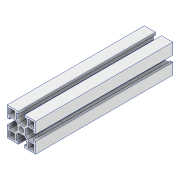
# Autodesk Inventor part: profile
Saved by Autodesk Inventor 2020 (Build 240168000, 168)
## iProperties
Created: 2020-09-09
Part Number: profile
Material: 알루미늄 6061
Document SubType Name: Modeling
Designer: 이호석
Mass: 133.418 g
Surface Area: 501.596 cm^2
Volume: 49.4139 cm^3
Density: 2.7 g/cm^3
Appearance: 알루미늄 - 평지
Author: 이호석
Autodesk Inventor part; units mm, degrees
ref_plane "YZ Plane" through (0, 0, 0) normal (1, 0, 0) x (0, 1, 0)
ref_plane "XZ Plane" through (0, 0, 0) normal (0, 1, 0) x (-1, 0, 0)
ref_plane "XY Plane" through (0, 0, 0) normal (0, 0, 1) x (1, 0, 0)
sketch "스케치1" plane through (0, 0, 0) normal (0, 0, 1) x (1, 0, 0)
  line L0 (15, -15) -> (-15, -15)
  line L1 (-15, -15) -> (-15, 15)
  line L2 (-15, 15) -> (15, 15)
  line L3 (15, 15) -> (15, -15)
  circle A0 centre (0, 0) radius 2.5
  line L4 (-3.15, -15) -> (3.15, -15)
  line L5 (-4.15, -15) -> (4.15, -15)
  line L6 (3.15, -15) -> (3.15, -12.5)
  line L7 (-3.15, -12.5) -> (-3.15, -15)
  line L8 (-5.5, -12.5) -> (5.5, -12.5)
  line L9 (5.5, -12.5) -> (5.5, -6.9)
  line L10 (-5.5, -6.9) -> (-5.5, -12.5)
  line L11 (-5.5, -6.9) -> (-3, -4.4)
  line L12 (5.5, -6.9) -> (3, -4.4)
  line L13 (-3, -4.4) -> (3, -4.4)
  line L14 (-13.25, -13.25) -> (-7.25, -13.25)
  line L15 (-7.25, -13.25) -> (-7.25, -7.25)
  line L16 (-7.25, -7.25) -> (-13.25, -7.25)
  line L17 (-13.25, -7.25) -> (-13.25, -13.25)
  line L18 (0, 0) -> (-1, 0)
  line L19 (0, 0) -> (0, -1)
  line L20 (13.25, -13.25) -> (7.25, -13.25)
  line L21 (7.25, -13.25) -> (7.25, -7.25)
  line L22 (7.25, -7.25) -> (13.25, -7.25)
  line L23 (13.25, -7.25) -> (13.25, -13.25)
  line L24 (-13.25, 13.25) -> (-7.25, 13.25)
  line L25 (-7.25, 13.25) -> (-7.25, 7.25)
  line L26 (-7.25, 7.25) -> (-13.25, 7.25)
  line L27 (-13.25, 7.25) -> (-13.25, 13.25)
  line L28 (13.25, 7.25) -> (13.25, 13.25)
  line L29 (13.25, 13.25) -> (7.25, 13.25)
  line L30 (7.25, 13.25) -> (7.25, 7.25)
  line L31 (7.25, 7.25) -> (13.25, 7.25)
  line L32 (6.9, 5.5) -> (4.4, 3)
  line L33 (12.5, 5.5) -> (6.9, 5.5)
  line L34 (15, -3.15) -> (15, 3.15)
  line L35 (15, -4.15) -> (15, 4.15)
  line L36 (15, 3.15) -> (12.5, 3.15)
  line L37 (12.5, -3.15) -> (15, -3.15)
  line L38 (12.5, -5.5) -> (12.5, 5.5)
  line L39 (6.9, -5.5) -> (12.5, -5.5)
  line L40 (4.4, -3) -> (4.4, 3)
  line L41 (6.9, -5.5) -> (4.4, -3)
  line L42 (-5.5, 6.9) -> (-3, 4.4)
  line L43 (-5.5, 12.5) -> (-5.5, 6.9)
  line L44 (3.15, 15) -> (-3.15, 15)
  line L45 (4.15, 15) -> (-4.15, 15)
  line L46 (-3.15, 15) -> (-3.15, 12.5)
  line L47 (3.15, 12.5) -> (3.15, 15)
  line L48 (5.5, 12.5) -> (-5.5, 12.5)
  line L49 (5.5, 6.9) -> (5.5, 12.5)
  line L50 (3, 4.4) -> (-3, 4.4)
  line L51 (5.5, 6.9) -> (3, 4.4)
  line L52 (-6.9, -5.5) -> (-4.4, -3)
  line L53 (-12.5, -5.5) -> (-6.9, -5.5)
  line L54 (-15, 3.15) -> (-15, -3.15)
  line L55 (-15, 4.15) -> (-15, -4.15)
  line L56 (-15, -3.15) -> (-12.5, -3.15)
  line L57 (-12.5, 3.15) -> (-15, 3.15)
  line L58 (-12.5, 5.5) -> (-12.5, -5.5)
  line L59 (-6.9, 5.5) -> (-12.5, 5.5)
  line L60 (-4.4, 3) -> (-4.4, -3)
  line L61 (-6.9, 5.5) -> (-4.4, 3)
  dimension "d0" = 30
  dimension "d1" = 30
  dimension "d4" = 6.3
  dimension "d20" = 6
  dimension "d21" = 6
  dimension "d22" = 1
  dimension "d23" = 1
  dimension "d26" = 360
  constraints: 124 end point, 12 symmetric about line, 11 point on line, 6 horizontal, 6 parallel, 3 perpendicular, 1 centre point, 1 coincident, 1 vertical, 93 other
  measures "d0" distance of L1.end L2.end
  measures "d1" distance of L0.end L1.end
  measures "d4" distance of L4.start L4.end
  measures "d20" distance of L16.end L15.end
  measures "d21" distance of L15.end L14.end
  measures "d22" distance of L18.start L18.end
  measures "d23" distance of L18.start L19.end
extrude "돌출1" add sketch "스케치1" along normal blind 144.5 contours L0 L6 L8 L9 L12 L13 L11 L10 L7 L1 L56 L58 L53 L52 L60 L61 L59 L57 L2 L46 L48 L43 L42 L50 L51 L49 L47 L3 L36 L38 L33 L32 L40 L41 L39 L37
